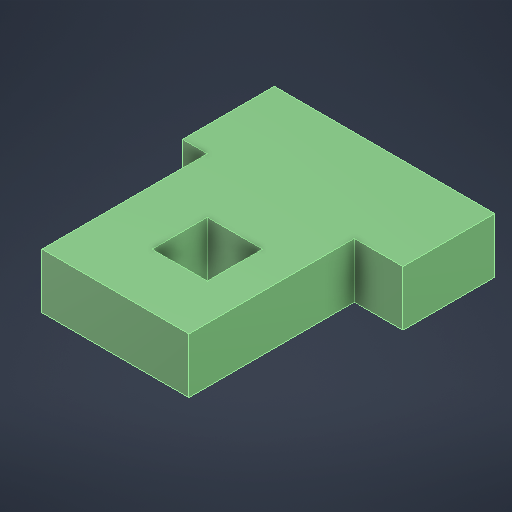
# Autodesk Inventor part: plug
Saved by Autodesk Inventor 2025.3 (Build 293356030, 356C)
## iProperties
Created: 2025-09-04
Part Number: plug
Material: 木材 (楓木)
Document SubType Name: Modeling
Designer: 陳泓任
Density: 0.67 g/cm^3
Appearance: 平滑 - 深森林綠
Author: 陳泓任
Autodesk Inventor part; units mm, degrees
ref_plane "YZ Plane" through (0, 0, 0) normal (1, 0, 0) x (0, 1, 0)
ref_plane "XZ Plane" through (0, 0, 0) normal (0, 1, 0) x (-1, 0, 0)
ref_plane "XY Plane" through (0, 0, 0) normal (0, 0, 1) x (1, 0, 0)
sketch "草圖1" plane through (0, 0, 0) normal (0, 1, 0) x (-1, 0, 0)
  line L0 (4, 11.5) -> (-4, 11.5)
  line L1 (-6.65, 2.5) -> (-6.65, -2.5)
  line L2 (5.35, -2.5) -> (5.35, 2.5)
  line L3 (5.35, 2.5) -> (4, 2.5)
  line L4 (-4, 2.5) -> (-6.65, 2.5)
  line L5 (-4, 11.5) -> (-4, 2.5)
  line L6 (0, 14.8546) -> (0, -17.157) construction
  line L7 (13.4413, 0) -> (-16.1444, 0) construction
  line L8 (4, 2.5) -> (4, 11.5)
  line L9 (5.35, -2.5) -> (-6.65, -2.5)
  line L10 (1, 5.5) -> (-2, 5.5)
  line L11 (-2, 5.5) -> (-2, 8.5)
  line L12 (-2, 8.5) -> (1, 8.5)
  line L13 (1, 8.5) -> (1, 5.5)
  line L14 (12.2, -7.6911) -> (12.2, 12.9035)
  point P0 (0, 0)
  point P1 (-6.65, 0)
  point P2 (5.35, 0)
  point P3 (0, 8.5)
  dimension "d0" = 8
  dimension "d3" = 5
  dimension "d5" = 12
  dimension "d9" = 9
  dimension "d13" = 1.35
  dimension "d17" = 28.4
  dimension "d18" = 3
  dimension "d19" = 3
  dimension "d20" = 3
  constraints: 30 end point, 7 perpendicular, 4 horizontal, 4 parallel, 4 point on line, 2 midpoint, 2 vertical, 1 collinear, 1 other
  measures "d0" distance of L0.start L0.end
  measures "d3" distance of L1.start L1.end
  measures "d5" distance between parallel lines of L1 L2
  measures "d9" distance of L0.end L4.start
  measures "d13" distance of L2.end L3.end
  measures "d17" diameter of L11 L14
  measures "d18" distance of L12.end L10.start
  measures "d19" distance between parallel lines of L10 L3
  measures "d20" distance between parallel lines of L8 L13
extrude "擠出1" add sketch "草圖1" along normal blind 3
